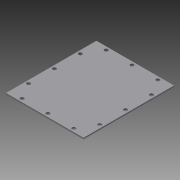
# Autodesk Inventor part: 090003-1
Saved by Autodesk Inventor 2015 (Build 190159000, 159)
## iProperties
Created: 2015-05-09
Part Number: 090003-1
Material: Generic
Document SubType Name: Modeling
Designer: Wesley
Density: 1 g/cm^3
Appearance: Default
Author: Wesley
Autodesk Inventor part; units mm, degrees
ref_plane "YZ Plane" through (0, 0, 0) normal (1, 0, 0) x (0, 1, 0)
ref_plane "XZ Plane" through (0, 0, 0) normal (0, 1, 0) x (-1, 0, 0)
ref_plane "XY Plane" through (0, 0, 0) normal (0, 0, 1) x (1, 0, 0)
sketch "Sketch1" plane through (0, 0, 0) normal (0, 1, 0) x (-1, 0, 0)
  line L0 (0, 0) -> (152.4, 0)
  line L1 (152.4, 0) -> (152.4, -177.8)
  line L2 (152.4, -177.8) -> (0, -177.8)
  line L3 (0, -177.8) -> (0, 0)
  dimension "d0" = 152.4
  dimension "d1" = 177.8
  constraints: 8 end point, 2 parallel, 1 horizontal, 1 perpendicular
  measures "d0" distance of L0.start L0.end
  measures "d1" distance of L0.end L1.end
extrude "Extrusion1" add sketch "Sketch1" along normal blind 2.54
sketch "Sketch2" plane through (0, 2.54, 0) normal (0, 1, 0) x (1, 0, 0)
  line L0 (-152.4, 0) -> (0, 0) projected
  line L1 (0, 0) -> (0, 177.8) projected
  line L2 (0, 177.8) -> (-152.4, 177.8) projected
  line L3 (-152.4, 177.8) -> (-152.4, 0) projected
  line L4 (-146.05, 6.35) -> (-6.35, 6.35) construction
  line L5 (-6.35, 6.35) -> (-6.35, 171.45) construction
  line L6 (-6.35, 171.45) -> (-146.05, 171.45) construction
  line L7 (-146.05, 171.45) -> (-146.05, 6.35) construction
  line L8 (-146.05, 171.45) -> (-127, 171.45) construction
  line L9 (-127, 171.45) -> (-127, 6.35) construction
  line L10 (-127, 6.35) -> (-146.05, 6.35) construction
  line L11 (-146.05, 6.35) -> (-146.05, 171.45) construction
  line L12 (-76.2, 6.35) -> (-127, 6.35) construction
  line L13 (-127, 6.35) -> (-127, 171.45) construction
  line L14 (-127, 171.45) -> (-76.2, 171.45) construction
  line L15 (-76.2, 171.45) -> (-76.2, 6.35) construction
  line L16 (-25.4, 6.35) -> (-6.35, 6.35) construction
  line L17 (-6.35, 6.35) -> (-6.35, 171.45) construction
  line L18 (-6.35, 171.45) -> (-25.4, 171.45) construction
  line L19 (-25.4, 171.45) -> (-25.4, 6.35) construction
  line L20 (0, 0) -> (0, 177.8) construction
  line L21 (-152.4, 0) -> (0, 0) construction
  line L22 (0, 0) -> (0, 12.7) construction
  line L23 (0, 12.7) -> (-152.4, 12.7) construction
  line L24 (-152.4, 12.7) -> (-152.4, 0) construction
  line L25 (-152.4, 177.8) -> (0, 177.8) construction
  line L26 (0, 177.8) -> (0, 165.1) construction
  line L27 (0, 165.1) -> (-152.4, 165.1) construction
  line L28 (-152.4, 165.1) -> (-152.4, 177.8) construction
  line L29 (-146.05, 38.1) -> (-6.35, 38.1) construction
  line L30 (-6.35, 38.1) -> (-6.35, 12.7) construction
  line L31 (-6.35, 12.7) -> (-146.05, 12.7) construction
  line L32 (-146.05, 12.7) -> (-146.05, 38.1) construction
  line L33 (-146.05, 38.1) -> (-6.35, 38.1) construction
  line L34 (-6.35, 38.1) -> (-6.35, 88.9) construction
  line L35 (-6.35, 88.9) -> (-146.05, 88.9) construction
  line L36 (-146.05, 88.9) -> (-146.05, 38.1) construction
  line L37 (-6.35, 88.9) -> (-146.05, 88.9) construction
  line L38 (-146.05, 88.9) -> (-146.05, 139.7) construction
  line L39 (-146.05, 139.7) -> (-6.35, 139.7) construction
  line L40 (-6.35, 139.7) -> (-6.35, 88.9) construction
  line L41 (-146.05, 139.7) -> (-6.35, 139.7) construction
  line L42 (-6.35, 139.7) -> (-6.35, 165.1) construction
  line L43 (-6.35, 165.1) -> (-146.05, 165.1) construction
  line L44 (-146.05, 165.1) -> (-146.05, 139.7) construction
  point P0 (-146.05, 88.9)
  dimension "d4" = 6.35
  dimension "d5" = 25.4
  dimension "d6" = 25.4
  dimension "d7" = 50.8
  dimension "d8" = 12.7
  dimension "d9" = 12.7
  dimension "d10" = 25.4
  dimension "d11" = 25.4
  dimension "d12" = 76.2
  constraints: 80 end point, 18 parallel, 10 point on line, 9 horizontal, 9 perpendicular, 6 coincident, 3 midpoint, 3 other
  measures "d4" distance between parallel lines of L3 L7
  measures "d5" distance from line of L3 L9.end
  measures "d6" distance from line of L1 L16.start
  measures "d7" distance of L12.start L16.start
  measures "d8" distance of L22.end L21.end
  measures "d9" distance of L25.end L26.end
  measures "d10" distance from line of L23 L29.start
  measures "d11" distance from line of L27 L38.end
  measures "d12" distance from line of L27 point (-146.05, 88.9)
hole "Hole1" at (-127, 2.54, -6.35) at (-76.2, 2.54, -6.35) at (-25.4, 2.54, -6.35) at (-127, 2.54, -171.45) at (-76.2, 2.54, -171.45) at (-25.4, 2.54, -171.45) at (-146.05, 2.54, -38.1) at (-146.05, 2.54, -88.9) at (-146.05, 2.54, -139.7) at (-6.35, 2.54, -38.1) at (-6.35, 2.54, -88.9) at (-6.35, 2.54, -139.7) direction (0, -1, 0) diameter 7.112 end through all
body "Solid1"
